Autodesk Inventor part; units mm, degrees
(part 2 of 2)
  spline S191 degree 2 poles (11.6445, 100.2631) (11.8831, 99.9981) (12.133, 99.4869) (12.133, 99.1991) knots 0 0 0 1 2 2 2
  spline S192 degree 2 poles (12.133, 99.1991) (12.133, 98.6841) (11.4514, 98.101) (10.8039, 98.101) knots 0 0 0 1 2 2 2
  line L240 (10.8039, 98.101) -> (8.5282, 98.101)
  spline S193 degree 2 poles (8.8993, 95.3179) (8.8463, 95.3898) (8.657, 95.6322) (8.6002, 95.7458) knots 0 0 0 1 2 2 2
  spline S194 degree 2 poles (8.6002, 95.7458) (8.5169, 95.901) (8.4298, 96.1926) (8.4298, 96.4576) knots 0 0 0 1 2 2 2
  spline S195 degree 2 poles (8.4298, 96.4576) (8.4298, 96.6735) (8.5926, 97.0635) (8.7403, 97.2112) knots 0 0 0 1 2 2 2
  spline S196 degree 2 poles (8.7403, 97.2112) (8.8841, 97.3513) (9.3082, 97.5217) (9.543, 97.5217) knots 0 0 0 1 2 2 2
  spline S197 degree 2 poles (9.543, 97.5217) (9.9065, 97.5217) (10.4215, 97.2149) (10.5692, 96.8817) knots 0 0 0 1 2 2 2
  spline S198 degree 2 poles (10.5692, 96.8817) (10.7055, 96.5864) (10.8077, 95.7836) (10.8342, 95.3179) knots 0 0 0 1 2 2 2
  line L241 (10.8342, 95.3179) -> (10.9478, 95.3179)
  spline S199 degree 2 poles (10.9478, 95.3179) (11.1523, 95.3179) (11.406, 95.4428) (11.4779, 95.5564) knots 0 0 0 1 2 2 2
  spline S200 degree 2 poles (11.4779, 95.5564) (11.5499, 95.67) (11.5953, 95.9957) (11.5953, 96.1699) knots 0 0 0 1 2 2 2
  spline S201 degree 2 poles (11.5953, 96.1699) (11.5953, 96.3743) (11.4741, 96.9272) (11.3568, 97.2036) knots 0 0 0 1 2 2 2
  line L242 (11.3568, 97.2036) -> (11.3568, 97.2377)
  line L243 (11.3568, 97.2377) -> (11.9588, 97.2377)
  spline S202 degree 2 poles (11.9588, 97.2377) (12.0043, 97.0748) (12.1178, 96.4652) (12.1178, 96.1661) knots 0 0 0 1 2 2 2
  spline S203 degree 2 poles (12.1178, 96.1661) (12.1178, 95.8026) (12.0043, 95.3065) (11.8566, 95.1096) knots 0 0 0 1 2 2 2
  spline S204 degree 2 poles (11.8566, 95.1096) (11.7127, 94.9165) (11.2545, 94.7272) (10.9251, 94.7272) knots 0 0 0 1 2 2 2
  line L244 (10.9251, 94.7272) -> (8.5282, 94.7272)
  line L245 (8.5282, 94.7272) -> (8.5282, 95.3179)
  line L246 (8.5282, 95.3179) -> (8.8993, 95.3179)
  line L247 (9.3915, 95.3179) -> (10.3647, 95.3179)
  spline S205 degree 2 poles (10.3647, 95.3179) (10.3457, 95.5299) (10.2814, 96.1699) (10.2208, 96.3705) knots 0 0 0 1 2 2 2
  spline S206 degree 2 poles (10.2208, 96.3705) (10.1488, 96.6053) (9.8497, 96.912) (9.5847, 96.912) knots 0 0 0 1 2 2 2
  spline S207 degree 2 poles (9.5847, 96.912) (9.2817, 96.912) (8.975, 96.5712) (8.975, 96.2456) knots 0 0 0 1 2 2 2
  spline S208 degree 2 poles (8.975, 96.2456) (8.975, 95.9692) (9.2136, 95.5148) (9.3915, 95.3179) knots 0 0 0 1 2 2 2
  spline S209 degree 2 poles (10.3382, 90.9596) (9.4786, 90.9596) (8.4298, 91.7926) (8.4298, 92.4212) knots 0 0 0 1 2 2 2
  spline S210 degree 2 poles (8.4298, 92.4212) (8.4298, 92.7052) (8.5699, 93.1103) (8.691, 93.3072) knots 0 0 0 1 2 2 2
  line L248 (8.691, 93.3072) -> (8.5282, 93.3451)
  line L249 (8.5282, 93.3451) -> (8.5282, 93.8979)
  line L250 (8.5282, 93.8979) -> (13.4091, 93.8979)
  line L251 (13.4091, 93.8979) -> (13.4091, 93.3072)
  line L252 (13.4091, 93.3072) -> (11.6672, 93.3072)
  spline S211 degree 2 poles (11.6672, 93.3072) (11.8679, 93.0838) (12.133, 92.5651) (12.133, 92.2357) knots 0 0 0 1 2 2 2
  spline S212 degree 2 poles (12.133, 92.2357) (12.133, 91.6412) (11.1826, 90.9596) (10.3382, 90.9596) knots 0 0 0 1 2 2 2
  spline S213 degree 2 poles (10.2927, 91.5692) (10.9213, 91.5692) (11.5726, 91.9517) (11.5726, 92.3758) knots 0 0 0 1 2 2 2
  spline S214 degree 2 poles (11.5726, 92.3758) (11.5726, 92.6143) (11.3454, 93.1066) (11.1712, 93.3072) knots 0 0 0 1 2 2 2
  line L253 (11.1712, 93.3072) -> (9.1606, 93.3072)
  spline S215 degree 2 poles (9.1606, 93.3072) (9.0508, 93.0838) (8.9599, 92.7393) (8.9599, 92.5348) knots 0 0 0 1 2 2 2
  spline S216 degree 2 poles (8.9599, 92.5348) (8.9599, 92.0842) (9.5998, 91.5692) (10.2927, 91.5692) knots 0 0 0 1 2 2 2
  line L254 (8.5282, 89.7441) -> (8.5282, 90.3348)
  line L255 (8.5282, 90.3348) -> (13.4091, 90.3348)
  line L256 (13.4091, 90.3348) -> (13.4091, 89.7441)
  line L257 (13.4091, 89.7441) -> (8.5282, 89.7441)
  spline S217 degree 2 poles (8.4487, 87.3548) (8.4487, 88.1954) (9.3915, 89.1193) (10.2624, 89.1193) knots 0 0 0 1 2 2 2
  spline S218 degree 2 poles (10.2624, 89.1193) (11.1182, 89.1193) (12.133, 88.2219) (12.133, 87.4987) knots 0 0 0 1 2 2 2
  spline S219 degree 2 poles (12.133, 87.4987) (12.133, 87.1731) (11.9437, 86.6694) (11.743, 86.4839) knots 0 0 0 1 2 2 2
  spline S220 degree 2 poles (11.743, 86.4839) (11.5423, 86.2946) (10.963, 86.0939) (10.5426, 86.0939) knots 0 0 0 1 2 2 2
  line L258 (10.5426, 86.0939) -> (10.2208, 86.0939)
  line L259 (10.2208, 86.0939) -> (10.2208, 88.5211)
  spline S221 degree 2 poles (10.2208, 88.5211) (9.6112, 88.5211) (8.9637, 87.9076) (8.9637, 87.3624) knots 0 0 0 1 2 2 2
  spline S222 degree 2 poles (8.9637, 87.3624) (8.9637, 87.1693) (9.0508, 86.7944) (9.1189, 86.6429) knots 0 0 0 1 2 2 2
  spline S223 degree 2 poles (9.1189, 86.6429) (9.1946, 86.4839) (9.3272, 86.2643) (9.3878, 86.1923) knots 0 0 0 1 2 2 2
  line L260 (9.3878, 86.1923) -> (9.3878, 86.1583)
  line L261 (9.3878, 86.1583) -> (8.744, 86.1583)
  spline S224 degree 2 poles (8.744, 86.1583) (8.7024, 86.2605) (8.5812, 86.571) (8.5471, 86.6922) knots 0 0 0 1 2 2 2
  spline S225 degree 2 poles (8.5471, 86.6922) (8.4979, 86.8626) (8.4487, 87.1428) (8.4487, 87.3548) knots 0 0 0 1 2 2 2
  spline S226 degree 2 poles (10.6714, 86.6694) (10.9099, 86.677) (11.2583, 86.7755) (11.3757, 86.8701) knots 0 0 0 1 2 2 2
  spline S227 degree 2 poles (11.3757, 86.8701) (11.5082, 86.9724) (11.6483, 87.2942) (11.6483, 87.5328) knots 0 0 0 1 2 2 2
  spline S228 degree 2 poles (11.6483, 87.5328) (11.6483, 87.7675) (11.5082, 88.097) (11.3719, 88.2333) knots 0 0 0 1 2 2 2
  spline S229 degree 2 poles (11.3719, 88.2333) (11.2318, 88.3658) (10.8948, 88.5021) (10.6714, 88.5211) knots 0 0 0 1 2 2 2
  line L262 (10.6714, 88.5211) -> (10.6714, 86.6694)
  line L263 (8.5282, 84.5793) -> (8.5282, 85.329)
  line L264 (8.5282, 85.329) -> (9.4218, 85.329)
  line L265 (9.4218, 85.329) -> (9.4218, 84.5793)
  line L266 (9.4218, 84.5793) -> (8.5282, 84.5793)
  spline S230 degree 2 poles (8.4487, 82.1559) (8.4487, 82.5194) (8.6721, 83.1215) (8.8993, 83.3373) knots 0 0 0 1 2 2 2
  spline S231 degree 2 poles (8.8993, 83.3373) (9.1227, 83.5531) (9.8118, 83.7917) (10.2738, 83.7917) knots 0 0 0 1 2 2 2
  spline S232 degree 2 poles (10.2738, 83.7917) (10.7358, 83.7917) (11.4098, 83.5456) (11.637, 83.3373) knots 0 0 0 1 2 2 2
  spline S233 degree 2 poles (11.637, 83.3373) (11.8679, 83.129) (12.1141, 82.5118) (12.1141, 82.1559) knots 0 0 0 1 2 2 2
  spline S234 degree 2 poles (12.1141, 82.1559) (12.1141, 81.8681) (11.9512, 81.3304) (11.8452, 81.1222) knots 0 0 0 1 2 2 2
  line L267 (11.8452, 81.1222) -> (11.1826, 81.1222)
  line L268 (11.1826, 81.1222) -> (11.1826, 81.1563)
  spline S235 degree 2 poles (11.1826, 81.1563) (11.2356, 81.2206) (11.3719, 81.4175) (11.4438, 81.5576) knots 0 0 0 1 2 2 2
  spline S236 degree 2 poles (11.4438, 81.5576) (11.5044, 81.6826) (11.5991, 82.0158) (11.5991, 82.1673) knots 0 0 0 1 2 2 2
  spline S237 degree 2 poles (11.5991, 82.1673) (11.5991, 82.6254) (10.9062, 83.182) (10.2738, 83.182) knots 0 0 0 1 2 2 2
  spline S238 degree 2 poles (10.2738, 83.182) (9.6566, 83.182) (8.9637, 82.6444) (8.9637, 82.1673) knots 0 0 0 1 2 2 2
  spline S239 degree 2 poles (8.9637, 82.1673) (8.9637, 81.8795) (9.2022, 81.3569) (9.3878, 81.1563) knots 0 0 0 1 2 2 2
  line L269 (9.3878, 81.1563) -> (9.3878, 81.1222)
  line L270 (9.3878, 81.1222) -> (8.7251, 81.1222)
  spline S240 degree 2 poles (8.7251, 81.1222) (8.6835, 81.2093) (8.5661, 81.4743) (8.5396, 81.5803) knots 0 0 0 1 2 2 2
  spline S241 degree 2 poles (8.5396, 81.5803) (8.4941, 81.7318) (8.4487, 81.9704) (8.4487, 82.1559) knots 0 0 0 1 2 2 2
  spline S242 degree 2 poles (10.2814, 77.7029) (9.3953, 77.7029) (8.4298, 78.5549) (8.4298, 79.2668) knots 0 0 0 1 2 2 2
  spline S243 degree 2 poles (8.4298, 79.2668) (8.4298, 79.9976) (9.4256, 80.8344) (10.2814, 80.8344) knots 0 0 0 1 2 2 2
  spline S244 degree 2 poles (10.2814, 80.8344) (11.1599, 80.8344) (12.133, 79.9711) (12.133, 79.2668) knots 0 0 0 1 2 2 2
  spline S245 degree 2 poles (12.133, 79.2668) (12.133, 78.5549) (11.1636, 77.7029) (10.2814, 77.7029) knots 0 0 0 1 2 2 2
  spline S246 degree 2 poles (10.2814, 78.3126) (10.963, 78.3126) (11.6256, 78.8086) (11.6256, 79.2668) knots 0 0 0 1 2 2 2
  spline S247 degree 2 poles (11.6256, 79.2668) (11.6256, 79.7249) (10.963, 80.2248) (10.2814, 80.2248) knots 0 0 0 1 2 2 2
  spline S248 degree 2 poles (10.2814, 80.2248) (9.6187, 80.2248) (8.9372, 79.7249) (8.9372, 79.2668) knots 0 0 0 1 2 2 2
  spline S249 degree 2 poles (8.9372, 79.2668) (8.9372, 78.8124) (9.6074, 78.3126) (10.2814, 78.3126) knots 0 0 0 1 2 2 2
  line L271 (8.5282, 74.4011) -> (8.5282, 74.9918)
  line L272 (8.5282, 74.9918) -> (8.8841, 74.9918)
  spline S250 degree 2 poles (8.8841, 74.9918) (8.7706, 75.1281) (8.6191, 75.3288) (8.5547, 75.4651) knots 0 0 0 1 2 2 2
  spline S251 degree 2 poles (8.5547, 75.4651) (8.4941, 75.59) (8.4298, 75.8589) (8.4298, 76.0369) knots 0 0 0 1 2 2 2
  spline S252 degree 2 poles (8.4298, 76.0369) (8.4298, 76.3246) (8.6683, 76.8093) (8.8993, 76.9797) knots 0 0 0 1 2 2 2
  spline S253 degree 2 poles (8.8993, 76.9797) (9.1303, 77.1501) (9.8118, 77.3394) (10.2549, 77.3394) knots 0 0 0 1 2 2 2
  spline S254 degree 2 poles (10.2549, 77.3394) (10.7168, 77.3394) (11.3908, 77.1009) (11.6445, 76.8926) knots 0 0 0 1 2 2 2
  spline S255 degree 2 poles (11.6445, 76.8926) (11.8717, 76.6995) (12.133, 76.158) (12.133, 75.8589) knots 0 0 0 1 2 2 2
  spline S256 degree 2 poles (12.133, 75.8589) (12.133, 75.5976) (12.0156, 75.2076) (11.8944, 74.9918) knots 0 0 0 1 2 2 2
  line L273 (11.8944, 74.9918) -> (13.4091, 74.9918)
  line L274 (13.4091, 74.9918) -> (13.4091, 74.4011)
  line L275 (13.4091, 74.4011) -> (8.5282, 74.4011)
  line L276 (9.3802, 74.9918) -> (11.406, 74.9918)
  spline S257 degree 2 poles (11.406, 74.9918) (11.512, 75.2114) (11.5915, 75.5598) (11.5915, 75.7604) knots 0 0 0 1 2 2 2
  spline S258 degree 2 poles (11.5915, 75.7604) (11.5915, 76.2148) (10.9099, 76.7298) (10.2662, 76.7298) knots 0 0 0 1 2 2 2
  spline S259 degree 2 poles (10.2662, 76.7298) (9.6452, 76.7298) (8.9902, 76.336) (8.9902, 75.9005) knots 0 0 0 1 2 2 2
  spline S260 degree 2 poles (8.9902, 75.9005) (8.9902, 75.6696) (9.2022, 75.2) (9.3802, 74.9918) knots 0 0 0 1 2 2 2
  line L277 (8.5282, 72.9433) -> (8.5282, 73.534)
  line L278 (8.5282, 73.534) -> (12.0345, 73.534)
  line L279 (12.0345, 73.534) -> (12.0345, 72.9433)
  line L280 (12.0345, 72.9433) -> (8.5282, 72.9433)
  line L281 (12.6177, 72.9016) -> (12.6177, 73.5718)
  line L282 (12.6177, 73.5718) -> (13.2311, 73.5718)
  line L283 (13.2311, 73.5718) -> (13.2311, 72.9016)
  line L284 (13.2311, 72.9016) -> (12.6177, 72.9016)
  line L285 (8.5282, 69.3233) -> (8.5282, 69.914)
  line L286 (8.5282, 69.914) -> (10.5275, 69.914)
  spline S261 degree 2 poles (10.5275, 69.914) (10.7698, 69.914) (11.1864, 69.9595) (11.3113, 70.0276) knots 0 0 0 1 2 2 2
  spline S262 degree 2 poles (11.3113, 70.0276) (11.4438, 70.0996) (11.5726, 70.3571) (11.5726, 70.5767) knots 0 0 0 1 2 2 2
  spline S263 degree 2 poles (11.5726, 70.5767) (11.5726, 70.7963) (11.3378, 71.262) (11.1485, 71.4854) knots 0 0 0 1 2 2 2
  line L287 (11.1485, 71.4854) -> (8.5282, 71.4854)
  line L288 (8.5282, 71.4854) -> (8.5282, 72.0761)
  line L289 (8.5282, 72.0761) -> (12.0345, 72.0761)
  line L290 (12.0345, 72.0761) -> (12.0345, 71.4854)
  line L291 (12.0345, 71.4854) -> (11.6445, 71.4854)
  spline S264 degree 2 poles (11.6445, 71.4854) (11.8831, 71.2204) (12.133, 70.7092) (12.133, 70.4214) knots 0 0 0 1 2 2 2
  spline S265 degree 2 poles (12.133, 70.4214) (12.133, 69.9065) (11.4514, 69.3233) (10.8039, 69.3233) knots 0 0 0 1 2 2 2
  line L292 (10.8039, 69.3233) -> (8.5282, 69.3233)
  spline S266 degree 2 poles (7.9678, 68.3691) (7.9413, 68.3085) (7.858, 68.0776) (7.8239, 67.9299) knots 0 0 0 1 2 2 2
  spline S267 degree 2 poles (7.8239, 67.9299) (7.7823, 67.7671) (7.733, 67.4906) (7.733, 67.3278) knots 0 0 0 1 2 2 2
  spline S268 degree 2 poles (7.733, 67.3278) (7.733, 67.0552) (7.8769, 66.6765) (8.0057, 66.5705) knots 0 0 0 1 2 2 2
  spline S269 degree 2 poles (8.0057, 66.5705) (8.1344, 66.4683) (8.4714, 66.3888) (8.6872, 66.3888) knots 0 0 0 1 2 2 2
  line L293 (8.6872, 66.3888) -> (8.994, 66.3888)
  spline S270 degree 2 poles (8.994, 66.3888) (8.7857, 66.6273) (8.5888, 67.0855) (8.5888, 67.4301) knots 0 0 0 1 2 2 2
  spline S271 degree 2 poles (8.5888, 67.4301) (8.5888, 68.0283) (9.4786, 68.7364) (10.3155, 68.7364) knots 0 0 0 1 2 2 2
  spline S272 degree 2 poles (10.3155, 68.7364) (10.7509, 68.7364) (11.4249, 68.4903) (11.6635, 68.2858) knots 0 0 0 1 2 2 2
  spline S273 degree 2 poles (11.6635, 68.2858) (11.8869, 68.0889) (12.133, 67.5474) (12.133, 67.2597) knots 0 0 0 1 2 2 2
  spline S274 degree 2 poles (12.133, 67.2597) (12.133, 66.987) (12.0043, 66.5895) (11.8869, 66.3888) knots 0 0 0 1 2 2 2
  line L294 (11.8869, 66.3888) -> (12.0345, 66.3547)
  line L295 (12.0345, 66.3547) -> (12.0345, 65.7981)
  line L296 (12.0345, 65.7981) -> (8.9296, 65.7981)
  spline S275 degree 2 poles (8.9296, 65.7981) (8.036, 65.7981) (7.2029, 66.5743) (7.2029, 67.3733) knots 0 0 0 1 2 2 2
  spline S276 degree 2 poles (7.2029, 67.3733) (7.2029, 67.6308) (7.2862, 68.1684) (7.3544, 68.3994) knots 0 0 0 1 2 2 2
  line L297 (7.3544, 68.3994) -> (7.9678, 68.3994)
  line L298 (7.9678, 68.3994) -> (7.9678, 68.3691)
  line L299 (9.4786, 66.3888) -> (11.406, 66.3888)
  spline S277 degree 2 poles (11.406, 66.3888) (11.512, 66.6084) (11.6029, 66.9795) (11.6029, 67.165) knots 0 0 0 1 2 2 2
  spline S278 degree 2 poles (11.6029, 67.165) (11.6029, 67.6118) (10.944, 68.1268) (10.3268, 68.1268) knots 0 0 0 1 2 2 2
  spline S279 degree 2 poles (10.3268, 68.1268) (9.7437, 68.1268) (9.1341, 67.7368) (9.1341, 67.2975) knots 0 0 0 1 2 2 2
  spline S280 degree 2 poles (9.1341, 67.2975) (9.1341, 67.0666) (9.3158, 66.5819) (9.4786, 66.3888) knots 0 0 0 1 2 2 2
  spline S281 degree 2 poles (8.4601, 63.8821) (8.4601, 64.363) (9.0091, 64.9044) (9.6036, 64.9044) knots 0 0 0 1 2 2 2
  line L300 (9.6036, 64.9044) -> (11.5461, 64.9044)
  line L301 (11.5461, 64.9044) -> (11.5461, 65.302)
  line L302 (11.5461, 65.302) -> (12.0345, 65.302)
  line L303 (12.0345, 65.302) -> (12.0345, 64.9044)
  line L304 (12.0345, 64.9044) -> (13.0418, 64.9044)
  line L305 (13.0418, 64.9044) -> (13.0418, 64.3137)
  line L306 (13.0418, 64.3137) -> (12.0345, 64.3137)
  line L307 (12.0345, 64.3137) -> (12.0345, 63.227)
  line L308 (12.0345, 63.227) -> (11.5461, 63.227)
  line L309 (11.5461, 63.227) -> (11.5461, 64.3137)
  line L310 (11.5461, 64.3137) -> (9.8762, 64.3137)
  spline S282 degree 2 poles (9.8762, 64.3137) (9.6112, 64.3137) (9.3196, 64.2948) (9.1946, 64.2304) knots 0 0 0 1 2 2 2
  spline S283 degree 2 poles (9.1946, 64.2304) (9.0848, 64.1774) (8.975, 63.9389) (8.975, 63.7344) knots 0 0 0 1 2 2 2
  spline S284 degree 2 poles (8.975, 63.7344) (8.975, 63.5905) (9.0621, 63.3217) (9.0886, 63.2611) knots 0 0 0 1 2 2 2
  line L311 (9.0886, 63.2611) -> (9.0886, 63.227)
  line L312 (9.0886, 63.227) -> (8.5585, 63.227)
  spline S285 degree 2 poles (8.5585, 63.227) (8.5131, 63.3936) (8.4601, 63.7344) (8.4601, 63.8821) knots 0 0 0 1 2 2 2
  line L313 (11.4022, 60.9324) -> (11.4022, 60.9627)
  spline S286 degree 2 poles (11.4022, 60.9627) (11.4211, 61.0308) (11.4287, 61.1785) (11.4287, 61.2807) knots 0 0 0 1 2 2 2
  spline S287 degree 2 poles (11.4287, 61.2807) (11.4287, 61.5193) (11.2204, 61.9888) (11.016, 62.2009) knots 0 0 0 1 2 2 2
  line L314 (11.016, 62.2009) -> (8.5282, 62.2009)
  line L315 (8.5282, 62.2009) -> (8.5282, 62.7916)
  line L316 (8.5282, 62.7916) -> (12.0345, 62.7916)
  line L317 (12.0345, 62.7916) -> (12.0345, 62.2009)
  line L318 (12.0345, 62.2009) -> (11.512, 62.2009)
  spline S288 degree 2 poles (11.512, 62.2009) (11.7998, 61.879) (12.0345, 61.3981) (12.0345, 61.1709) knots 0 0 0 1 2 2 2
  spline S289 degree 2 poles (12.0345, 61.1709) (12.0345, 61.08) (12.027, 60.9892) (12.0156, 60.9324) knots 0 0 0 1 2 2 2
  line L319 (12.0156, 60.9324) -> (11.4022, 60.9324)
  line L320 (8.5282, 59.8721) -> (8.5282, 60.4628)
  line L321 (8.5282, 60.4628) -> (12.0345, 60.4628)
  line L322 (12.0345, 60.4628) -> (12.0345, 59.8721)
  line L323 (12.0345, 59.8721) -> (8.5282, 59.8721)
  line L324 (12.6177, 59.8305) -> (12.6177, 60.5007)
  line L325 (12.6177, 60.5007) -> (13.2311, 60.5007)
  line L326 (13.2311, 60.5007) -> (13.2311, 59.8305)
  line L327 (13.2311, 59.8305) -> (12.6177, 59.8305)
  spline S290 degree 2 poles (8.4487, 57.6116) (8.4487, 57.9751) (8.6721, 58.5771) (8.8993, 58.793) knots 0 0 0 1 2 2 2
  spline S291 degree 2 poles (8.8993, 58.793) (9.1227, 59.0088) (9.8118, 59.2474) (10.2738, 59.2474) knots 0 0 0 1 2 2 2
  spline S292 degree 2 poles (10.2738, 59.2474) (10.7358, 59.2474) (11.4098, 59.0012) (11.637, 58.793) knots 0 0 0 1 2 2 2
  spline S293 degree 2 poles (11.637, 58.793) (11.8679, 58.5847) (12.1141, 57.9675) (12.1141, 57.6116) knots 0 0 0 1 2 2 2
  spline S294 degree 2 poles (12.1141, 57.6116) (12.1141, 57.3238) (11.9512, 56.7861) (11.8452, 56.5779) knots 0 0 0 1 2 2 2
  line L328 (11.8452, 56.5779) -> (11.1826, 56.5779)
  line L329 (11.1826, 56.5779) -> (11.1826, 56.6119)
  spline S295 degree 2 poles (11.1826, 56.6119) (11.2356, 56.6763) (11.3719, 56.8732) (11.4438, 57.0133) knots 0 0 0 1 2 2 2
  spline S296 degree 2 poles (11.4438, 57.0133) (11.5044, 57.1383) (11.5991, 57.4715) (11.5991, 57.6229) knots 0 0 0 1 2 2 2
  spline S297 degree 2 poles (11.5991, 57.6229) (11.5991, 58.0811) (10.9062, 58.6377) (10.2738, 58.6377) knots 0 0 0 1 2 2 2
  spline S298 degree 2 poles (10.2738, 58.6377) (9.6566, 58.6377) (8.9637, 58.1) (8.9637, 57.6229) knots 0 0 0 1 2 2 2
  spline S299 degree 2 poles (8.9637, 57.6229) (8.9637, 57.3352) (9.2022, 56.8126) (9.3878, 56.6119) knots 0 0 0 1 2 2 2
  line L330 (9.3878, 56.6119) -> (9.3878, 56.5779)
  line L331 (9.3878, 56.5779) -> (8.7251, 56.5779)
  spline S300 degree 2 poles (8.7251, 56.5779) (8.6835, 56.6649) (8.5661, 56.93) (8.5396, 57.036) knots 0 0 0 1 2 2 2
  spline S301 degree 2 poles (8.5396, 57.036) (8.4941, 57.1875) (8.4487, 57.426) (8.4487, 57.6116) knots 0 0 0 1 2 2 2
  line L332 (8.5282, 53.1359) -> (8.5282, 53.9121)
  line L333 (8.5282, 53.9121) -> (10.2208, 55.2147)
  line L334 (10.2208, 55.2147) -> (9.9936, 55.4495)
  line L335 (9.9936, 55.4495) -> (8.5282, 55.4495)
  line L336 (8.5282, 55.4495) -> (8.5282, 56.0402)
  line L337 (8.5282, 56.0402) -> (13.4091, 56.0402)
  line L338 (13.4091, 56.0402) -> (13.4091, 55.4495)
  line L339 (13.4091, 55.4495) -> (10.554, 55.4495)
  line L340 (10.554, 55.4495) -> (12.0345, 54.0636)
  line L341 (12.0345, 54.0636) -> (12.0345, 53.329)
  line L342 (12.0345, 53.329) -> (10.5692, 54.7679)
  line L343 (10.5692, 54.7679) -> (8.5282, 53.1359)
  spline S302 degree 2 poles (8.4449, 51.8939) (8.4449, 52.2461) (8.6342, 52.8557) (8.7403, 53.0564) knots 0 0 0 1 2 2 2
  line L344 (8.7403, 53.0564) -> (9.4029, 53.0564)
  line L345 (9.4029, 53.0564) -> (9.4029, 53.0261)
  spline S303 degree 2 poles (9.4029, 53.0261) (9.3423, 52.9504) (9.1984, 52.7459) (9.1189, 52.5755) knots 0 0 0 1 2 2 2
  spline S304 degree 2 poles (9.1189, 52.5755) (9.047, 52.4278) (8.9409, 52.0643) (8.9409, 51.8712) knots 0 0 0 1 2 2 2
  spline S305 degree 2 poles (8.9409, 51.8712) (8.9409, 51.7311) (9.0053, 51.4092) (9.0583, 51.3335) knots 0 0 0 1 2 2 2
  spline S306 degree 2 poles (9.0583, 51.3335) (9.1303, 51.2237) (9.2931, 51.1252) (9.4597, 51.1252) knots 0 0 0 1 2 2 2
  spline S307 degree 2 poles (9.4597, 51.1252) (9.668, 51.1252) (9.8838, 51.3524) (9.9557, 51.644) knots 0 0 0 1 2 2 2
  spline S308 degree 2 poles (9.9557, 51.644) (9.9822, 51.7576) (10.058, 52.1211) (10.0996, 52.2764) knots 0 0 0 1 2 2 2
  spline S309 degree 2 poles (10.0996, 52.2764) (10.217, 52.6777) (10.7017, 53.0412) (11.0463, 53.0412) knots 0 0 0 1 2 2 2
  spline S310 degree 2 poles (11.0463, 53.0412) (11.5234, 53.0412) (12.1178, 52.3256) (12.1178, 51.7349) knots 0 0 0 1 2 2 2
  spline S311 degree 2 poles (12.1178, 51.7349) (12.1178, 51.4433) (11.974, 50.8526) (11.8641, 50.6519) knots 0 0 0 1 2 2 2
  line L346 (11.8641, 50.6519) -> (11.2318, 50.6519)
  line L347 (11.2318, 50.6519) -> (11.2318, 50.6822)
  spline S312 degree 2 poles (11.2318, 50.6822) (11.4136, 50.9094) (11.6218, 51.4622) (11.6218, 51.7462) knots 0 0 0 1 2 2 2
  spline S313 degree 2 poles (11.6218, 51.7462) (11.6218, 52.0378) (11.3757, 52.4392) (11.1296, 52.4392) knots 0 0 0 1 2 2 2
  spline S314 degree 2 poles (11.1296, 52.4392) (10.9062, 52.4392) (10.6903, 52.2006) (10.6222, 51.9356) knots 0 0 0 1 2 2 2
  spline S315 degree 2 poles (10.6222, 51.9356) (10.5881, 51.8068) (10.5199, 51.4812) (10.4783, 51.3032) knots 0 0 0 1 2 2 2
  spline S316 degree 2 poles (10.4783, 51.3032) (10.3798, 50.917) (9.9292, 50.5232) (9.5392, 50.5232) knots 0 0 0 1 2 2 2
  spline S317 degree 2 poles (9.5392, 50.5232) (9.312, 50.5232) (8.9107, 50.7012) (8.763, 50.8753) knots 0 0 0 1 2 2 2
  spline S318 degree 2 poles (8.763, 50.8753) (8.6077, 51.0609) (8.4449, 51.5342) (8.4449, 51.8939) knots 0 0 0 1 2 2 2
  line L348 (12.0345, 47.2213) -> (7.237, 49.107)
  line L349 (7.237, 49.107) -> (7.237, 49.7394)
  line L350 (7.237, 49.7394) -> (8.6986, 49.1108)
  line L351 (8.6986, 49.1108) -> (12.0345, 50.3831)
  line L352 (12.0345, 50.3831) -> (12.0345, 49.7469)
  line L353 (12.0345, 49.7469) -> (9.437, 48.789)
  line L354 (9.437, 48.789) -> (12.0345, 47.8347)
  line L355 (12.0345, 47.8347) -> (12.0345, 47.2213)
  spline S319 degree 2 poles (8.4601, 45.7143) (8.4601, 46.1952) (9.0091, 46.7367) (9.6036, 46.7367) knots 0 0 0 1 2 2 2
  line L356 (9.6036, 46.7367) -> (11.5461, 46.7367)
  line L357 (11.5461, 46.7367) -> (11.5461, 47.1342)
  line L358 (11.5461, 47.1342) -> (12.0345, 47.1342)
  line L359 (12.0345, 47.1342) -> (12.0345, 46.7367)
  line L360 (12.0345, 46.7367) -> (13.0418, 46.7367)
  line L361 (13.0418, 46.7367) -> (13.0418, 46.146)
  line L362 (13.0418, 46.146) -> (12.0345, 46.146)
  line L363 (12.0345, 46.146) -> (12.0345, 45.0592)
  line L364 (12.0345, 45.0592) -> (11.5461, 45.0592)
  line L365 (11.5461, 45.0592) -> (11.5461, 46.146)
  line L366 (11.5461, 46.146) -> (9.8762, 46.146)
  spline S320 degree 2 poles (9.8762, 46.146) (9.6112, 46.146) (9.3196, 46.127) (9.1946, 46.0626) knots 0 0 0 1 2 2 2
  spline S321 degree 2 poles (9.1946, 46.0626) (9.0848, 46.0096) (8.975, 45.7711) (8.975, 45.5666) knots 0 0 0 1 2 2 2
  spline S322 degree 2 poles (8.975, 45.5666) (8.975, 45.4227) (9.0621, 45.1539) (9.0886, 45.0933) knots 0 0 0 1 2 2 2
  line L367 (9.0886, 45.0933) -> (9.0886, 45.0592)
  line L368 (9.0886, 45.0592) -> (8.5585, 45.0592)
  spline S323 degree 2 poles (8.5585, 45.0592) (8.5131, 45.2258) (8.4601, 45.5666) (8.4601, 45.7143) knots 0 0 0 1 2 2 2
  line L369 (8.5282, 43.7074) -> (8.5282, 44.4572)
  line L370 (8.5282, 44.4572) -> (9.4218, 44.4572)
  line L371 (9.4218, 44.4572) -> (9.4218, 43.7074)
  line L372 (9.4218, 43.7074) -> (8.5282, 43.7074)
  spline S324 degree 2 poles (8.4487, 41.284) (8.4487, 41.6475) (8.6721, 42.2496) (8.8993, 42.4654) knots 0 0 0 1 2 2 2
  spline S325 degree 2 poles (8.8993, 42.4654) (9.1227, 42.6813) (9.8118, 42.9198) (10.2738, 42.9198) knots 0 0 0 1 2 2 2
  spline S326 degree 2 poles (10.2738, 42.9198) (10.7358, 42.9198) (11.4098, 42.6737) (11.637, 42.4654) knots 0 0 0 1 2 2 2
  spline S327 degree 2 poles (11.637, 42.4654) (11.8679, 42.2572) (12.1141, 41.64) (12.1141, 41.284) knots 0 0 0 1 2 2 2
  spline S328 degree 2 poles (12.1141, 41.284) (12.1141, 40.9963) (11.9512, 40.4586) (11.8452, 40.2503) knots 0 0 0 1 2 2 2
  line L373 (11.8452, 40.2503) -> (11.1826, 40.2503)
  line L374 (11.1826, 40.2503) -> (11.1826, 40.2844)
  spline S329 degree 2 poles (11.1826, 40.2844) (11.2356, 40.3488) (11.3719, 40.5457) (11.4438, 40.6858) knots 0 0 0 1 2 2 2
  spline S330 degree 2 poles (11.4438, 40.6858) (11.5044, 40.8107) (11.5991, 41.1439) (11.5991, 41.2954) knots 0 0 0 1 2 2 2
  spline S331 degree 2 poles (11.5991, 41.2954) (11.5991, 41.7536) (10.9062, 42.3102) (10.2738, 42.3102) knots 0 0 0 1 2 2 2
  spline S332 degree 2 poles (10.2738, 42.3102) (9.6566, 42.3102) (8.9637, 41.7725) (8.9637, 41.2954) knots 0 0 0 1 2 2 2
  spline S333 degree 2 poles (8.9637, 41.2954) (8.9637, 41.0076) (9.2022, 40.4851) (9.3878, 40.2844) knots 0 0 0 1 2 2 2
  line L375 (9.3878, 40.2844) -> (9.3878, 40.2503)
  line L376 (9.3878, 40.2503) -> (8.7251, 40.2503)
  spline S334 degree 2 poles (8.7251, 40.2503) (8.6835, 40.3374) (8.5661, 40.6025) (8.5396, 40.7085) knots 0 0 0 1 2 2 2
  spline S335 degree 2 poles (8.5396, 40.7085) (8.4941, 40.8599) (8.4487, 41.0985) (8.4487, 41.284) knots 0 0 0 1 2 2 2
  spline S336 degree 2 poles (10.2814, 36.8311) (9.3953, 36.8311) (8.4298, 37.683) (8.4298, 38.3949) knots 0 0 0 1 2 2 2
  spline S337 degree 2 poles (8.4298, 38.3949) (8.4298, 39.1257) (9.4256, 39.9625) (10.2814, 39.9625) knots 0 0 0 1 2 2 2
  spline S338 degree 2 poles (10.2814, 39.9625) (11.1599, 39.9625) (12.133, 39.0992) (12.133, 38.3949) knots 0 0 0 1 2 2 2
  spline S339 degree 2 poles (12.133, 38.3949) (12.133, 37.683) (11.1636, 36.8311) (10.2814, 36.8311) knots 0 0 0 1 2 2 2
  spline S340 degree 2 poles (10.2814, 37.4407) (10.963, 37.4407) (11.6256, 37.9367) (11.6256, 38.3949) knots 0 0 0 1 2 2 2
  spline S341 degree 2 poles (11.6256, 38.3949) (11.6256, 38.8531) (10.963, 39.3529) (10.2814, 39.3529) knots 0 0 0 1 2 2 2
  spline S342 degree 2 poles (10.2814, 39.3529) (9.6187, 39.3529) (8.9372, 38.8531) (8.9372, 38.3949) knots 0 0 0 1 2 2 2
  spline S343 degree 2 poles (8.9372, 38.3949) (8.9372, 37.9405) (9.6074, 37.4407) (10.2814, 37.4407) knots 0 0 0 1 2 2 2
  line L377 (8.5282, 32.2494) -> (10.5578, 32.2494)
  spline S344 degree 2 poles (10.5578, 32.2494) (10.8001, 32.2494) (11.2129, 32.2872) (11.3265, 32.3478) knots 0 0 0 1 2 2 2
  spline S345 degree 2 poles (11.3265, 32.3478) (11.4514, 32.4084) (11.5726, 32.6394) (11.5726, 32.8401) knots 0 0 0 1 2 2 2
  spline S346 degree 2 poles (11.5726, 32.8401) (11.5726, 33.0218) (11.3492, 33.4383) (11.1371, 33.658) knots 0 0 0 1 2 2 2
  spline S347 degree 2 poles (11.1371, 33.658) (11.0841, 33.6542) (10.9364, 33.6466) (10.838, 33.6466) knots 0 0 0 1 2 2 2
  line L378 (10.838, 33.6466) -> (8.5282, 33.6466)
  line L379 (8.5282, 33.6466) -> (8.5282, 34.2373)
  line L380 (8.5282, 34.2373) -> (10.5578, 34.2373)
  spline S348 degree 2 poles (10.5578, 34.2373) (10.8001, 34.2373) (11.2129, 34.2752) (11.3265, 34.3358) knots 0 0 0 1 2 2 2
  spline S349 degree 2 poles (11.3265, 34.3358) (11.4514, 34.3963) (11.5726, 34.6273) (11.5726, 34.828) knots 0 0 0 1 2 2 2
  spline S350 degree 2 poles (11.5726, 34.828) (11.5726, 35.0173) (11.334, 35.4376) (11.1485, 35.6345) knots 0 0 0 1 2 2 2
  line L381 (11.1485, 35.6345) -> (8.5282, 35.6345)
  line L382 (8.5282, 35.6345) -> (8.5282, 36.2252)
  line L383 (8.5282, 36.2252) -> (12.0345, 36.2252)
  line L384 (12.0345, 36.2252) -> (12.0345, 35.6345)
  line L385 (12.0345, 35.6345) -> (11.6483, 35.6345)
  spline S351 degree 2 poles (11.6483, 35.6345) (11.8793, 35.4036) (12.133, 34.9492) (12.133, 34.6765) knots 0 0 0 1 2 2 2
  spline S352 degree 2 poles (12.133, 34.6765) (12.133, 34.366) (11.849, 33.8852) (11.5271, 33.7602) knots 0 0 0 1 2 2 2
  spline S353 degree 2 poles (11.5271, 33.7602) (11.8263, 33.4914) (12.133, 32.984) (12.133, 32.6886) knots 0 0 0 1 2 2 2
  spline S354 degree 2 poles (12.133, 32.6886) (12.133, 32.4614) (11.9929, 32.0903) (11.8339, 31.954) knots 0 0 0 1 2 2 2
  spline S355 degree 2 poles (11.8339, 31.954) (11.6748, 31.8139) (11.1977, 31.6587) (10.838, 31.6587) knots 0 0 0 1 2 2 2
  line L386 (10.838, 31.6587) -> (8.5282, 31.6587)
  line L387 (8.5282, 31.6587) -> (8.5282, 32.2494)
  point P0 (0, 2)
  constraints: 2 other
extrude "Extrusion18" cut sketch "Sketch14" against normal blind 1.75
extrude "Extrusion19" add sketch "Sketch11" against normal up to surface (132 mm away) contours L0 A1 L14 L9 L1 L2 | L13 A0 L3 L11
sketch "Sketch12" plane through (-32.5, 0, 0) normal (0, 1, 0) x (1, 0, 0)
  line L0 (32.5, 2) -> (32.5, -122)
  line L1 (54.5, -122) -> (10.5, -122) projected
  line L2 (32.5, -60) -> (59.2, -60)
  line L3 (32.5, -60) -> (5.8, -60)
  line L4 (59.2, -60) -> (59.2, -27)
  line L5 (60.0149, -32) -> (60.0149, -21) projected
  line L6 (59.2, -60) -> (92.2, -60) construction
  line L7 (59.2, -60) -> (59.2, -93)
  line L8 (59.2, -93) -> (5.8, -93)
  line L9 (5.8, -93) -> (5.8, -27)
  line L10 (5.8, -27) -> (59.2, -27)
  line L11 (59.2, -27) -> (59.2, -93)
  line L12 (59.2, -27) -> (57.2, -27)
  line L13 (57.2, -27) -> (56.5, -24.0828)
  line L14 (56.5, -21) -> (56.5, -32) projected
  line L15 (56.5, -24.0828) -> (18.5, -24.0828)
  line L16 (18.5, -24.0828) -> (18.5, -27)
  line L17 (59.2, -27) -> (52.2, -27)
  circle A0 centre (52.2, -25.5828) radius 1.5
  circle A1 centre (23.2, -25.5828) radius 1.5
  line L18 (59.2, -93) -> (59.2, -79.2)
  circle A2 centre (57.7, -79.2) radius 1.5
  line L19 (5.8, -93) -> (5.8, -78)
  circle A3 centre (7.3, -78) radius 1.5
  point P0 (32.5, 0)
  point P1 (51.7085, -27)
  point P2 (52.6915, -27)
  point P3 (22.7085, -27)
  point P4 (23.6915, -27)
  dimension "d138" = 26.7
  dimension "d139" = 26.7
  dimension "d140" = 33
  dimension "d141" = 90
  dimension "d142" = 33
  dimension "d143" = 66
  dimension "d144" = 2
  dimension "d146" = 38
  dimension "d148" = 3
  dimension "d150" = 3
  dimension "d151" = 13.8
  dimension "d152" = 3
  dimension "d153" = 15
  dimension "d154" = 3
  constraints: 34 end point, 6 point on line, 4 centre point, 4 horizontal, 4 parallel, 3 perpendicular, 3 tangent, 2 midpoint, 1 vertical
  measures "d138" distance of L2.start L2.end
  measures "d139" distance of L2.start L3.end
  measures "d140" distance of L2.end L4.end
  measures "d141" angle of L6 L4
  measures "d142" distance of L2.end L7.end
  measures "d143" distance of L8.end L9.end
  measures "d144" distance of L10.end L12.end
  measures "d146" distance of L13.end L15.end
  measures "d148" diameter of A0
  measures "d150" diameter of A1
  measures "d151" distance of L7.end L18.end
  measures "d152" diameter of A2
  measures "d153" distance of L8.end L19.end
  measures "d154" diameter of A3
extrude "Extrusion17" cut sketch "Sketch12" along normal mid plane 10 contours A0 L10 | A1 L10 | A2 | A3 picked at (52.0841, -25.0688) picked at (23.6224, -26.0822)
sketch "Sketch15" plane through (34.2324, 24.7969, 132) normal (0, 0, 1) x (1, 0, 0)
  line L0 (-56.2324, -29.7969) -> (-56.2324, -24.7969) projected
  line L1 (-56.2324, -24.7969) -> (-56.2324, -22.7969)
  line L2 (-1.4524, -22.7969) -> (-67.0125, -22.7969) projected
  line L3 (-12.2324, -24.7969) -> (-12.2324, -29.7969) projected
  line L4 (-12.2324, -24.7969) -> (-12.2324, -22.7969)
  line L5 (-7.2324, -22.7969) -> (-67.0125, -22.7969) projected
  line L6 (-65.7912, -24.7969) -> (-7.2324, -24.7969) projected
  point P0 (-34.2324, -24.7969)
  constraints: 4 end point, 2 vertical, 1 point on line
extrude "Extrusion20" cut sketch "Sketch15" against normal blind 10
body "Solid2"
